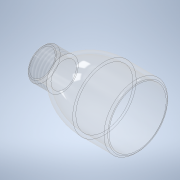
# Autodesk Inventor part: Outer
Saved by Autodesk Inventor 2021 (Build 250183000, 183)
## iProperties
Created: 2021-07-30
Part Number: Outer
Material: PET Plastic
Document SubType Name: Modeling
Designer: Shammy Haider
Density: 1.541 g/cm^3
Appearance: Polycarbonate - Clear
Author: Shammy Haider
Autodesk Inventor part; units mm, degrees
ref_plane "YZ Plane" through (0, 0, 0) normal (1, 0, 0) x (0, 1, 0)
ref_plane "XZ Plane" through (0, 0, 0) normal (0, 1, 0) x (-1, 0, 0)
ref_plane "XY Plane" through (0, 0, 0) normal (0, 0, 1) x (1, 0, 0)
sketch "Sketch1" plane through (0, 0, 0) normal (0, 0, 1) x (1, 0, 0)
  line L0 (-9.5356, 0) -> (8.6335, 0)
  line L1 (-9.7709, 2.5) -> (-6.6144, 2.5)
  arc A0 (0, 5) -> (-6.6144, 2.5) centre (0, -5) ccw
  line L2 (0, 0) -> (0, 8.0856)
  line L3 (0, 5) -> (5.2291, 5)
  line L4 (5.2291, 5) -> (5.2291, 0)
  line L5 (-9.7709, 0) -> (-9.7709, 2.5)
  dimension "d0" = 5
  dimension "d1" = 10
  dimension "d2" = 10
  dimension "d4" = 15
  constraints: 12 end point, 4 point on line, 3 horizontal, 2 perpendicular, 2 point on circle, 1 centre point, 1 tangent, 1 vertical
  measures "d0" diameter of L1 L0
  measures "d1" radius of A0
  measures "d2" diameter of L3 L0
  measures "d4" distance between parallel lines of L5 L4
surface revolve "RevolutionSrf1" sketch "Sketch1" angle 360 about axis through (-9.5356, 0, 0) along (1, 0, 0) shown yes curves L3 A0 L1
thicken "Thicken1" operation new thickness 0.5 both sides no extend neighbours no toward (0, -0.9967573, 0.0804666) faces at (-7.6666, 2.4919, -0.2012) (-2.3859, 4.3342, -1.8466) (3.486, 4.9353, -0.8021)
thread "Thread1" size "M5.5x0.5" class "6g" standard "ANSI Metric M Profile" length 160
fillet "Fillet1" radius 0.3 2 edges at (5.2291, -5, 0) (-9.7709, -2.5, 0)
body "Solid1"
body "Srf1"
